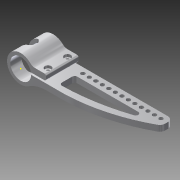
# Autodesk Inventor part: suporte-rodas-esq
Saved by Autodesk Inventor 2015 (Build 190159000, 159)
## iProperties
Created: 2016-08-10
Part Number: suporte-rodas-esq
Material: Aluminium AW-7020
Document SubType Name: Modeling
Designer: EriveltonDell
Density: 2.78 g/cm^3
Appearance: Polished - Small Pyramid Knurl
Mass: 207.794 g
Surface Area: 308.105 cm^2
Volume: 74.746 cm^3
Author: EriveltonDell
Autodesk Inventor part; units mm, degrees
ref_plane "YZ Plane" through (0, 0, 0) normal (1, 0, 0) x (0, 1, 0)
ref_plane "XZ Plane" through (0, 0, 0) normal (0, 1, 0) x (-1, 0, 0)
ref_plane "XY Plane" through (0, 0, 0) normal (0, 0, 1) x (1, 0, 0)
sketch "Sketch1" plane through (0, 0, 0) normal (0, 1, 0) x (-1, 0, 0)
  arc A0 (-16, 0) -> (-15.7162, 3) centre (0, 0) ccw
  arc A1 (-11.6822, -17.4507) -> (-14.7951, 14.9032) centre (0, 0) ccw
  line L0 (-16, 0) -> (-184, 0)
  line L1 (-184, 0) -> (-184, -9)
  line L2 (-184, -9) -> (-39.4968, -9)
  arc A2 (-11.6822, -17.4507) -> (-39.4968, -9) centre (-39.4968, -59) ccw
  line L3 (-39, 12) -> (-39, 3)
  line L4 (0, 0) -> (0, 3)
  line L5 (-15.7162, 3) -> (-39, 3)
  line L6 (-39, 3) -> (-39, 12)
  line L7 (-39, 12) -> (-21.8403, 12)
  arc A3 (-21.8403, 12) -> (-14.7951, 14.9032) centre (-21.8403, 22) ccw
  point P0 (-18.9737, -9)
  point P1 (-17.2337, 12)
  dimension "d0" = 32
  dimension "d1" = 42
  dimension "d2" = 168
  dimension "d3" = 9
  dimension "d4" = 50
  dimension "d7" = 3
  dimension "d8" = 39
  dimension "d9" = 9
  dimension "d10" = 3
  dimension "d11" = 39
  dimension "d12" = 10
  constraints: 16 end point, 10 point on circle, 4 centre point, 4 perpendicular, 4 tangent, 2 coincident, 2 point on line, 1 horizontal, 1 vertical
  measures "d0" diameter of A0
  measures "d1" diameter of A1
  measures "d2" distance of L0.start L0.end
  measures "d3" distance of L0.end L1.end
  measures "d4" radius of A2
  measures "d7" distance of L4.start L4.end
  measures "d8" distance of L3.end L4.end
  measures "d9" distance of L3.end L3.start
  measures "d10" distance from line of L0 L5.start
  measures "d11" distance from line of L4.start L3
  measures "d12" radius of A3
extrude "Extrusion1" add sketch "Sketch1" along normal blind 50
hole "Hole1" at (32, 10, 12) direction (0, 0, -1) diameter 5.5 end through all counterbore diameter 10 counterbore depth 4
hole "Hole2" at (32, 40, 12) direction (0, 0, -1) diameter 5.5 end through all counterbore diameter 10 counterbore depth 4
sketch "Sketch3" plane through (16, 0, 0) normal (0, 0, 1) x (1, 0, 0)
  point P0 (-16, 0)
fillet "Fillet1" radius 2.5 2 edges at (39, 25, 12) (39, 25, 3)
sketch "Sketch4" plane through (0, 0, 0) normal (0, 1, 0) x (-1, 0, 0)
  point P0 (0, 0)
sketch "Sketch5" plane through (0, 0, 0) normal (0, 0, 1) x (1, 0, 0)
  line L0 (0, 0) -> (0, 17)
  line L1 (14.7951, 50) -> (-21, 50) projected
  line L2 (-8, 17) -> (-40, 17)
  line L3 (-40, 17) -> (-40, 33)
  line L4 (-40, 33) -> (-8, 33)
  line L5 (0, 25) -> (0, 25)
  arc A0 (0, 25) -> (-8, 33) centre (-8, 25) ccw
  arc A1 (-8, 17) -> (0, 25) centre (-8, 25) ccw
  point P0 (11.6822, 50)
  point P1 (0, 33)
  dimension "d41" = 17
  dimension "d42" = 40
  dimension "d43" = 16
  dimension "d44" = 40
  dimension "d45" = 8
  constraints: 10 end point, 5 point on line, 4 point on circle, 4 tangent, 3 perpendicular, 2 centre point, 1 concentric
  measures "d41" distance of L0.start L0.end
  measures "d42" distance of L0.end L2.end
  measures "d43" distance of L2.end L3.end
  measures "d44" distance of L3.end point (0, 33)
  measures "d45" radius of A0
extrude "Extrusion3" cut sketch "Sketch5" along normal through all both and the other way through all
sketch "Sketch8" plane through (16, 0, 0) normal (0, 0, 1) x (1, 0, 0)
  line L0 (-16, 0) -> (-16, 50)
  line L1 (-32, 50) -> (0, 50) projected
  line L2 (-16, 50) -> (34, 50)
  line L3 (0, 50) -> (168, 50) projected
  line L4 (34, 50) -> (34, 33)
  line L5 (34, 33) -> (154, 33)
  line L6 (168, 0) -> (168, 50) projected
  line L7 (51.1, 0) -> (173.3862, 0) construction
  line L8 (34, 50) -> (38, 50)
  line L9 (38, 50) -> (38, 41.5)
  circle A0 centre (38, 41.5) radius 3.1
  circle A1 centre (48, 41.5) radius 3.1
  circle A2 centre (58, 41.5) radius 3.1
  circle A3 centre (68, 41.5) radius 3.1
  circle A4 centre (78, 41.5) radius 3.1
  circle A5 centre (88, 41.5) radius 3.1
  circle A6 centre (98, 41.5) radius 3.1
  circle A7 centre (108, 41.5) radius 3.1
  circle A8 centre (118, 41.5) radius 3.1
  circle A9 centre (128, 41.5) radius 3.1
  circle A10 centre (138, 41.5) radius 3.1
  circle A11 centre (148, 41.5) radius 3.1
  circle A12 centre (158, 41.5) radius 3.1
  arc A13 (34, 9.0247) -> (154, 33) centre (32.6984, 327.8368) ccw
  line L10 (34, 0) -> (168, 0)
  line L11 (168, 0) -> (168, 33)
  arc A14 (34, 0) -> (51.1, 0) centre (42.55, 253.8424) ccw
  line L12 (34, 9.0247) -> (34, 33)
  arc A15 (34, 0) -> (168, 33) centre (42.55, 253.8424) ccw
  point P0 (-0.2838, 50)
  dimension "d49" = 50
  dimension "d50" = 17
  dimension "d54" = 4
  dimension "d55" = 8.5
  dimension "d56" = 6.2
  dimension "d59" = 10
  dimension "d73" = 120
  dimension "d74" = 23.9753
  constraints: 21 end point, 16 centre point, 7 point on circle, 4 point on line, 2 horizontal, 2 perpendicular, 2 vertical, 1 coincident, 1 collinear, 1 midpoint, 24 other
  measures "d49" distance of L0.end L2.end
  measures "d50" distance of L2.end L4.end
  measures "d54" distance of L2.end L8.end
  measures "d55" distance of L8.end L9.end
  measures "d56" diameter of A0
  measures "d59" distance of A0.centre A1.centre
  measures "d73" distance of L4.end L5.end
  measures "d74" distance of L4.end L12.start
extrude "Extrusion4" cut sketch "Sketch8" against normal through all contours L5 A13 L12 | L10 A15 L6 | A0 | A1 | A2 | A3 | A4 | A5 | A6 | A7 | A8 | A9 | A10 | A11 | A12
fillet "Fillet2" radius 4 1 edges at (170, 33, -4.5)
fillet "Fillet3" radius 4 2 edges at (50, 33, -4.5) (50, 9.0247, -4.5)
fillet "Fillet4" radius 8 2 edges at (184, 50, -4.5) (184, 33, -4.5)
body "Solid1"
